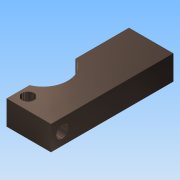
# Autodesk Inventor part: держатель шкива
Saved by Autodesk Inventor 2017 (Build 210142000, 142)
## iProperties
Part Number: держатель шкива
Material: Типовые
Document SubType Name: Modeling
Designer: Max
Mass: 3.97883 g
Surface Area: 21.5737 cm^2
Volume: 3.97883 cm^3
Density: 1 g/cm^3
Appearance: Оружейный металл — антик — полированный
Author: Max
Autodesk Inventor part; units mm, degrees
ref_plane "YZ Plane" through (0, 0, 0) normal (1, 0, 0) x (0, 1, 0)
ref_plane "XZ Plane" through (0, 0, 0) normal (0, 1, 0) x (-1, 0, 0)
ref_plane "XY Plane" through (0, 0, 0) normal (0, 0, 1) x (1, 0, 0)
sketch "Эскиз1" plane through (0, 0, 0) normal (0, 0, 1) x (1, 0, 0)
  line L0 (0, 0) -> (-14.5, 0)
  line L1 (-14.5, 0) -> (-14.5, 40)
  line L2 (-14.5, 40) -> (0, 40)
  line L3 (0, 40) -> (0, 0)
  circle A0 centre (-11.5, 4) radius 2
  arc A1 (-14.5, 7.5) -> (-14.5, 22.5) centre (-17.6022, 15) ccw
  dimension "d0" = 14.5
  dimension "d1" = 40
  dimension "d2" = 4
  dimension "d4" = 4
  dimension "d5" = 11.5
  dimension "d6" = 15
  dimension "d7" = 15
  constraints: 8 end point, 2 centre point, 2 parallel, 2 point on circle, 2 point on line, 1 horizontal, 1 perpendicular
  measures "d0" distance of L1.end L2.end
  measures "d1" distance between parallel lines of L0 L2
  measures "d2" diameter of A0
  measures "d4" distance from line of L0 A0.centre
  measures "d5" distance from line of L3 A0.centre
  measures "d6" distance from line of L0 A1.centre
  measures "d7" distance of A1.start A1.end
extrude "Выдавливание1" add sketch "Эскиз1" along normal mid plane 8 contours L0 L1 A1 L2 L3
sketch "Эскиз2" plane through (0, 0, 4) normal (1, 0, 0) x (0, 0, -1)
  circle A0 centre (4, 5.9) radius 2
  line L0 (4, 0) -> (4, 4.8588) construction
  line L1 (8, 0) -> (0, 0) projected
  dimension "d10" = 4
  dimension "d16" = 5.9
  constraints: 2 end point, 1 centre point, 1 vertical
  measures "d10" diameter of A0
  measures "d16" distance from line of L1 A0.centre
extrude "Выдавливание2" cut sketch "Эскиз2" against normal blind 5
sketch "Эскиз3" plane through (-14.5, 40, 4) normal (0, 1, 0) x (1, 0, 0)
  circle A0 centre (4.4, 4) radius 2
  line L0 (14.5, 4) -> (4.4, 4) construction
  line L1 (14.5, 8) -> (14.5, 0) projected
  dimension "d13" = 4
  dimension "d17" = 10.1
  constraints: 2 end point, 1 centre point, 1 horizontal
  measures "d13" diameter of A0
  measures "d17" distance from line of L1 L0.end
extrude "Выдавливание3" cut sketch "Эскиз3" against normal blind 5
